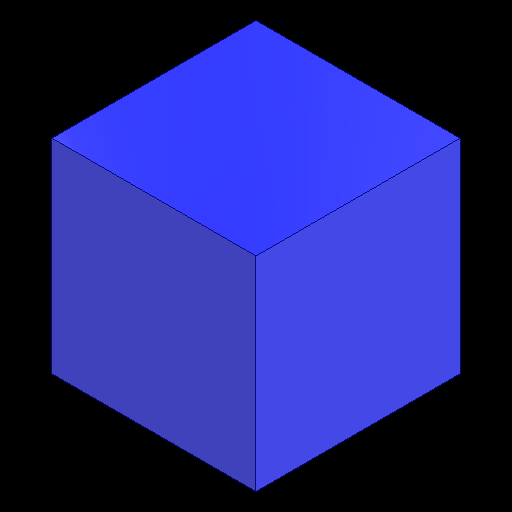
# Autodesk Inventor part: кубик
Saved by Autodesk Inventor 2025 (Build 290162000, 162)
## iProperties
Created: 2025-03-10
Part Number: кубик
Material: Типовые
Document SubType Name: Modeling
Designer: volko
Density: 1 g/cm^3
Appearance: Синий — малярная краска — глянцевая
Mass: 64 g
Surface Area: 96 cm^2
Volume: 64 cm^3
Author: volko
Autodesk Inventor part; units mm, degrees
ref_plane "YZ Plane" through (0, 0, 0) normal (1, 0, 0) x (0, 1, 0)
ref_plane "XZ Plane" through (0, 0, 0) normal (0, 1, 0) x (-1, 0, 0)
ref_plane "XY Plane" through (0, 0, 0) normal (0, 0, 1) x (1, 0, 0)
sketch "Эскиз1" plane through (0, 0, 0) normal (0, 1, 0) x (-1, 0, 0)
  line L0 (20, 20) -> (-20, 20)
  line L1 (-20, 20) -> (-20, -20)
  line L2 (-20, -20) -> (20, -20)
  line L3 (20, -20) -> (20, 20)
  line L4 (28, 0) -> (-28, 0) projected
  line L5 (0, -28) -> (0, 28) projected
  point P0 (0, 0)
  dimension "d2" = 40
  constraints: 8 end point, 2 parallel, 2 perpendicular, 1 horizontal, 2 other
  measures "d2" distance of L1.end L2.end
extrude "Выдавливание1" add sketch "Эскиз1" along normal blind 40
